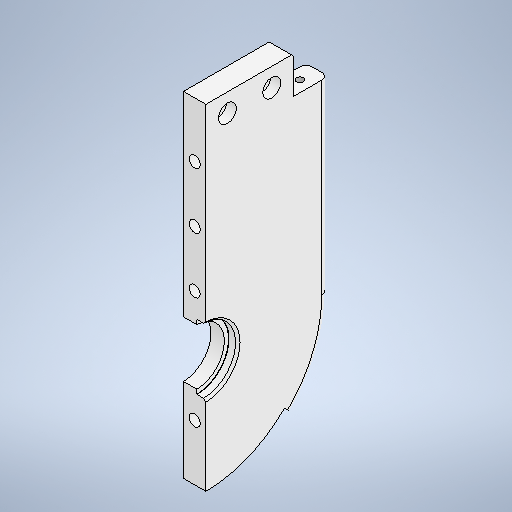
# Autodesk Inventor part: joint4_frame_support
Saved by Autodesk Inventor 2025.3 (Build 293356030, 356C)
## iProperties
Created: 2025-11-09
Part Number: joint4_frame_support
Material: PLA filament
Document SubType Name: Modeling
Designer: MSI
Mass: 82.4617 g
Surface Area: 191.265 cm^2
Volume: 68.7181 cm^3
Density: 1.2 g/cm^3
Appearance: 일반
Author: MSI
Autodesk Inventor part; units mm, degrees
ref_plane "YZ Plane" through (0, 0, 0) normal (1, 0, 0) x (0, 1, 0)
ref_plane "XZ Plane" through (0, 0, 0) normal (0, 1, 0) x (-1, 0, 0)
sketch "스케치1" plane through (0, 0, 0) normal (1, 0, 0) x (0, 1, 0)
  circle A0 centre (0, 0) radius 55
  line L0 (0, 55) -> (99.7, 55)
  line L1 (99.7, 55) -> (99.7, -55)
  line L2 (99.7, -55) -> (0, -55)
  line L3 (0, -55) -> (0, 55)
  point P0 (0, 55)
  point P1 (0, -55)
  dimension "d0" = 110
  dimension "d1" = 110
  dimension "d2" = 99.7
  constraints: 8 end point, 2 coincident, 2 parallel, 1 centre point, 1 horizontal, 1 midpoint, 1 perpendicular
  measures "d0" diameter of A0
  measures "d1" distance of L0.end L1.end
  measures "d2" distance of L1.end L2.end
extrude "돌출1" add sketch "스케치1" along normal mid plane 10
sketch "스케치2" plane through (-5, 0, 55) normal (0, 0, 1) x (1, 0, 0)
  line L0 (0, 99.7) -> (0, 0) projected
  line L1 (10, 99.7) -> (10, 0) projected
  line L2 (0, 99.7) -> (10, 99.7)
  line L3 (10, 99.7) -> (10, 83.2)
  line L4 (10, 83.2) -> (0, 83.2)
  line L5 (0, 83.2) -> (0, 99.7)
  point P0 (5, 0)
  point P1 (10, 99.7)
  point P2 (0, 83.2)
  dimension "d5" = 16.5
  constraints: 8 end point, 2 parallel, 1 horizontal, 1 perpendicular, 1 point on line
  measures "d5" distance between parallel lines of L2 L4
extrude "돌출2" cut sketch "스케치2" against normal blind 15.5
mirror "미러1" about plane through (0, 0, 0) normal (0, 0, 1) of "돌출2"
sketch "스케치3" plane through (5, 0, 0) normal (1, 0, 0) x (0, 0, -1)
  arc A0 (-55, 0) -> (55, 0) centre (0, 0) ccw projected
  constraints: 1 coincident
hole "구멍1" at (5, 0, 0) direction (-1, 0, 0) diameter 25 end through all counterbore diameter 29 counterbore depth 4
fillet "모깎기1" radius 0.1 1 edges at (1, 0, 14.5)
sketch "스케치4" plane through (5, 0, 0) normal (1, 0, 0) x (0, 0, -1)
  line L0 (-29.625, 91.45) -> (29.625, 91.45) construction
  line L1 (-39.5, 99.7) -> (-39.5, 83.2) projected
  line L2 (39.5, 99.7) -> (-39.5, 99.7) projected
  point P0 (0, 0)
  point P1 (-39.5, 91.45)
  point P2 (0, 91.45)
  point P3 (0, 99.7)
  point P4 (9.875, 91.45)
  point P5 (-9.875, 91.45)
  dimension "d16" = 19.75
  dimension "d17" = 19.75
  dimension "d18" = 59.25
  constraints: 3 midpoint, 3 point on line, 2 coincident, 2 end point, 1 horizontal, 1 vertical alignment
  measures "d16" distance of point (-9.875, 91.45) point (-29.625, 91.45)
  measures "d17" distance of point (9.875, 91.45) point (29.625, 91.45)
  measures "d18" distance of L0.start L0.end
hole "구멍2" at (5, 91.45, 29.625) at (5, 91.45, -29.625) at (5, 91.45, -9.875) at (5, 91.45, 9.875) direction (-1, 0, 0) diameter 4.5 end through all counterbore diameter 8 counterbore depth 4.4 clearance for "Socket Head Cap Screw ISO 4762" size "M4" standard "ISO"
sketch "스케치5" plane through (-5, 83.2, 55) normal (0, 1, 0) x (1, 0, 0)
  line L0 (5, 102.25) -> (5, 7.75)
  line L1 (0, 94.5) -> (0, 110) projected
  line L2 (0, 0) -> (0, 15.5) projected
  line L3 (0, 110) -> (10, 110) projected
  point P0 (5, 55)
  point P1 (0, 102.25)
  point P2 (0, 7.75)
  point P3 (5, 110)
  constraints: 3 midpoint, 2 end point, 2 horizontal alignment, 1 point on line, 1 vertical
hole "구멍3" at (0, 83.2, -47.25) at (0, 83.2, 47.25) direction (0, -1, 0) diameter 3.242 depth 11 tip angle 118 thread size "M4x0.7" class "6H" standard "ISO Metric profile"
chamfer "모따기1" distance 1 angle 45 3 edges at (0, 99.7, 39.5) (0, 99.7, -39.5) (5, 0, 14.5)
fillet "모깎기2" radius 3 6 edges at (5, 41.6, -55) (5, 41.6, 55) (5, -55, 0) (-5, 41.6, 55) (-5, 41.6, -55) (-5, -55, 0)
sketch "스케치6" plane through (0, 0, 0) normal (1, 0, 0) x (0, 1, 0)
  arc A0 (0, 55) -> (0, -55) centre (0, 0) ccw projected
  line L0 (-38.8909, 38.8909) -> (0, 0)
  line L1 (0, 0) -> (-55, 0)
  arc A1 (0, 50) -> (0, -50) centre (0, 0) ccw
  point P0 (-50, 0)
  point P1 (-35.3553, 35.3553)
  dimension "d37" = 5
  dimension "d38" = 45
  constraints: 4 end point, 4 point on circle, 1 centre point, 1 horizontal
  measures "d37" radial gap between concentric circles of A0 A1
  measures "d38" angle of L0 L1
extrude "돌출3" cut sketch "스케치6" along normal through all both and the other way through all contours L0 A1 L1 A0
sketch "스케치7" plane through (0, 0, 0) normal (1, 0, 0) x (0, 1, 0)
  line L0 (0, 0) -> (-40.9576, 28.6788)
  arc A0 (-35.3553, 35.3553) -> (-50, 0) centre (0, 0) ccw projected
  arc A1 (-55, 0) -> (0, -55) centre (0, 0) ccw projected
  line L1 (-55, 0) -> (0, 0)
  dimension "d41" = 35
  constraints: 4 end point, 1 horizontal, 1 point on circle
  measures "d41" angle of L1 L0
ref_plane "작업 평면1" through (0, -40.9576, 28.6788) normal (0, -0.819152, 0.5735764) x (1, 0, 0)
sketch "스케치8" plane through (0, -40.9576, 28.6788) normal (0, -0.819152, 0.5735764) x (1, 0, 0)
  point P0 (0, 0)
  point P1 (0, 0)
  constraints: 1 coincident
hole "구멍4" at (0, -40.9576, 28.6788) direction (0, 0.819152, -0.5735764) diameter 3.242 depth 12 tip angle 118 thread size "M4x0.7" class "6H" standard "ISO Metric profile"
mirror "미러2" about plane through (0, 0, 0) normal (0, 0, 1) of "구멍4", "돌출3"
sketch "스케치9" plane through (0, 0, 0) normal (1, 0, 0) x (0, 1, 0)
  line L0 (126.0553, -0.25) -> (-78.4769, -0.25)
  line L1 (-78.4769, -0.25) -> (-78.4769, -164.2979)
  line L2 (-78.4769, -164.2979) -> (126.0553, -164.2979)
  line L3 (126.0553, -164.2979) -> (126.0553, -0.25)
  point P0 (0, 0)
  dimension "d63" = 0.25
  constraints: 8 end point, 2 parallel, 1 horizontal, 1 perpendicular
  measures "d63" distance from line of L0 point (0, 0)
extrude "돌출4" cut sketch "스케치9" along normal through all both and the other way through all keep common part
sketch "스케치10" plane through (5, 99.7, -0.25) normal (0, 0, 1) x (1, 0, 0)
  line L0 (-5, -124.7) -> (-5, -24.7)
  point P0 (-5, -99.7)
  point P1 (-5, -74.7)
  point P2 (-5, -49.7)
  dimension "d52" = 100
  dimension "d53" = 25
  dimension "d54" = 25
  dimension "d55" = 25
  constraints: 2 coincident, 2 end point, 2 point on line, 1 midpoint, 1 vertical
  measures "d52" distance of L0.start L0.end
  measures "d53" distance of point (-5, -99.7) point (-5, -124.7)
  measures "d54" distance of point (-5, -99.7) point (-5, -74.7)
  measures "d55" distance of point (-5, -74.7) point (-5, -49.7)
hole "구멍5" at (0, -25, -0.25) at (0, 25, -0.25) at (0, 50, -0.25) at (0, 75, -0.25) direction (0, 0, -1) diameter 5 depth 10 tip angle 118
equation "\"d17\" = d16"
equation "\"d18\" = 3 * d16"
equation "\"d52\" = 4 * d53"
equation "\"d54\" = d53"
equation "\"d55\" = d54"
